Autodesk Inventor part; units mm, degrees
(part 4 of 5)
sketch "Эскиз44" plane through (1.5, 0, 0) normal (1, 0, 0) x (0, 0, -1)
  line L0 (40, 27.152) -> (40, 3) projected
  arc A0 (37, 0) -> (40, 3) centre (37, 3) ccw projected
  line L1 (37, 0) -> (-7, 0) projected
  arc A1 (-10, 3) -> (-7, 0) centre (-7, 3) ccw projected
  line L2 (-10, 3) -> (-10, 160) projected
  arc A2 (-7, 163) -> (-10, 160) centre (-7, 160) ccw projected
  line L3 (-7, 163) -> (37, 163) projected
  arc A3 (40, 160) -> (37, 163) centre (37, 160) ccw projected
  line L4 (40, 160) -> (40, 111.152) projected
  arc A4 (40, 111.152) -> (42, 109.152) centre (42, 111.152) ccw projected
  line L5 (42, 109.152) -> (54, 109.152) projected
  arc A5 (56, 107.152) -> (54, 109.152) centre (54, 107.152) ccw projected
  line L6 (56, 107.152) -> (56, 31.152) projected
  arc A6 (54, 29.152) -> (56, 31.152) centre (54, 31.152) ccw projected
  line L7 (54, 29.152) -> (42, 29.152) projected
  circle A7 centre (383.6, 368.9) radius 1.625 projected
  circle A8 centre (-13.6, 369) radius 1.625 projected
  circle A9 centre (383.6, 1.1) radius 1.625 projected
  circle A10 centre (-13.6, 1.1) radius 1.625 projected
  circle A11 centre (379.0468, 185.0848) radius 1.625 projected
  circle A12 centre (-9.0468, 185.0848) radius 1.625 projected
  circle A13 centre (379, 228) radius 1.625 projected
  circle A14 centre (-9, 228) radius 1.625 projected
  arc A15 (314.8984, 369.1946) -> (314.8984, 366.8054) centre (313.7968, 368) ccw projected
  arc A16 (314.8984, 366.8054) -> (314.8984, 369.1946) centre (316, 368) ccw projected
  arc A17 (297.8984, 229.1946) -> (297.8984, 226.8054) centre (296.7968, 228) ccw projected
  arc A18 (297.8984, 226.8054) -> (297.8984, 229.1946) centre (299, 228) ccw projected
  circle A19 centre (54, 228) radius 1.625 projected
  circle A20 centre (71, 142) radius 1.625 projected
  circle A21 centre (71, 2.0002) radius 1.625 projected
  circle A22 centre (54, 2.0002) radius 1.625 projected
  circle A23 centre (71, 368) radius 1.625 projected
  circle A24 centre (71, 228) radius 1.625 projected
  arc A25 (314.8984, 143.1946) -> (314.8984, 140.8054) centre (313.7968, 142) ccw projected
  arc A26 (314.8984, 140.8054) -> (314.8984, 143.1946) centre (316, 142) ccw projected
  arc A27 (314.8984, 229.1946) -> (314.8984, 226.8054) centre (313.7968, 228) ccw projected
  arc A28 (314.8984, 226.8054) -> (314.8984, 229.1946) centre (316, 228) ccw projected
  circle A29 centre (183.175, 129.0059) radius 1.85 projected
  arc A30 (297.8984, 369.1946) -> (297.8984, 366.8054) centre (296.7968, 368) ccw projected
  arc A31 (297.8984, 366.8054) -> (297.8984, 369.1946) centre (299, 368) ccw projected
  arc A32 (314.8984, 3.1948) -> (314.8984, 0.8056) centre (313.7968, 2.0002) ccw projected
  arc A33 (314.8984, 0.8056) -> (314.8984, 3.1948) centre (316, 2.0002) ccw projected
  circle A34 centre (54, 142) radius 1.625 projected
  circle A35 centre (54, 368) radius 1.625 projected
  arc A36 (297.8984, 3.1948) -> (297.8984, 0.8056) centre (296.7968, 2.0002) ccw projected
  arc A37 (297.8984, 0.8056) -> (297.8984, 3.1948) centre (299, 2.0002) ccw projected
  arc A38 (297.8984, 143.1946) -> (297.8984, 140.8054) centre (296.7968, 142) ccw projected
  arc A39 (297.8984, 140.8054) -> (297.8984, 143.1946) centre (299, 142) ccw projected
  arc A40 (185, 193.309) -> (185, 192.7028) centre (183.175, 193.0059) ccw projected
  line L8 (185, 193.309) -> (185, 192.7028) projected
  line L9 (14.5, 247.5001) -> (35, 247.5001) projected
  arc A41 (38, 244.5001) -> (35, 247.5001) centre (35, 244.5001) ccw projected
  line L10 (38, 244.5001) -> (38, 185.5001) projected
  arc A42 (35, 182.5001) -> (38, 185.5001) centre (35, 185.5001) ccw projected
  line L11 (35, 182.5001) -> (14.5, 182.5001) projected
  arc A43 (11.5, 185.5001) -> (14.5, 182.5001) centre (14.5, 185.5001) ccw projected
  line L12 (11.5, 185.5001) -> (11.5, 244.5001) projected
  arc A44 (14.5, 247.5001) -> (11.5, 244.5001) centre (14.5, 244.5001) ccw projected
  line L13 (358.5, 244.5001) -> (358.5, 185.5001) projected
  arc A45 (355.5, 182.5001) -> (358.5, 185.5001) centre (355.5, 185.5001) ccw projected
  line L14 (355.5, 182.5001) -> (335, 182.5001) projected
  arc A46 (332, 185.5001) -> (335, 182.5001) centre (335, 185.5001) ccw projected
  line L15 (332, 185.5001) -> (332, 244.5001) projected
  arc A47 (335, 247.5001) -> (332, 244.5001) centre (335, 244.5001) ccw projected
  line L16 (335, 247.5001) -> (355.5, 247.5001) projected
  arc A48 (358.5, 244.5001) -> (355.5, 247.5001) centre (355.5, 244.5001) ccw projected
  line L17 (98.825, 226.3849) -> (98.825, 137.3849) projected
  arc A49 (95.825, 134.3849) -> (98.825, 137.3849) centre (95.825, 137.3849) ccw projected
  line L18 (95.825, 134.3849) -> (87.825, 134.3849) projected
  arc A50 (84.825, 137.3849) -> (87.825, 134.3849) centre (87.825, 137.3849) ccw projected
  line L19 (84.825, 137.3849) -> (84.825, 226.3849) projected
  arc A51 (87.825, 229.3849) -> (84.825, 226.3849) centre (87.825, 226.3849) ccw projected
  line L20 (87.825, 229.3849) -> (95.825, 229.3849) projected
  arc A52 (98.825, 226.3849) -> (95.825, 229.3849) centre (95.825, 226.3849) ccw projected
  circle A53 centre (124.375, 129.0059) radius 2 projected
  circle A54 centre (124.375, 193.0059) radius 2 projected
  circle A55 centre (217.25, 312.9941) radius 2.1 projected
  circle A56 centre (152.75, 57.0059) radius 2.1 projected
  circle A57 centre (152.75, 118.0059) radius 2.1 projected
  circle A58 centre (152.75, 312.9941) radius 2.1 projected
  circle A59 centre (217.25, 251.9941) radius 2.1 projected
  circle A60 centre (217.25, 57.0059) radius 2.1 projected
  circle A61 centre (217.25, 118.0059) radius 2.1 projected
  circle A62 centre (152.75, 251.9941) radius 2.1 projected
  line L21 (165, 44) -> (165, 8) projected
  arc A63 (162, 5) -> (165, 8) centre (162, 8) ccw projected
  line L22 (162, 5) -> (96, 5) projected
  arc A64 (93, 8) -> (96, 5) centre (96, 8) ccw projected
  line L23 (93, 8) -> (93, 44) projected
  arc A65 (96, 47) -> (93, 44) centre (96, 44) ccw projected
  line L24 (96, 47) -> (162, 47) projected
  arc A66 (165, 44) -> (162, 47) centre (162, 44) ccw projected
  circle A67 centre (319.1128, 165.0002) radius 2.1 projected
  circle A68 centre (287, 56.343) radius 2.1 projected
  circle A69 centre (50.8872, 165.0002) radius 2.1 projected
  circle A70 centre (173.9908, 56.343) radius 2.1 projected
  circle A71 centre (135.25, 60) radius 2.1 projected
  circle A72 centre (103, 60) radius 2.1 projected
  line L25 (226.25, 270.0041) -> (226.25, 298.657) projected
  arc A73 (228.25, 300.657) -> (226.25, 298.657) centre (228.25, 298.657) ccw projected
  line L26 (228.25, 300.657) -> (268.3252, 300.657) projected
  arc A74 (269.4885, 297.03) -> (268.3252, 300.657) centre (268.3252, 298.657) ccw projected
  line L27 (269.4885, 297.03) -> (229.4132, 268.3772) projected
  arc A75 (226.25, 270.0041) -> (229.4132, 268.3772) centre (228.25, 270.0041) ccw projected
  arc A76 (235.9248, 170.343) -> (234.7615, 166.7161) centre (235.9248, 168.343) ccw projected
  line L28 (235.9248, 170.343) -> (276, 170.343) projected
  arc A77 (278, 168.343) -> (276, 170.343) centre (276, 168.343) ccw projected
  line L29 (278, 168.343) -> (278, 139.6902) projected
  arc A78 (274.8368, 138.0633) -> (278, 139.6902) centre (276, 139.6902) ccw projected
  line L30 (274.8368, 138.0633) -> (234.7615, 166.7161) projected
  arc A79 (94, 106.343) -> (92, 104.343) centre (94, 104.343) ccw projected
  line L31 (94, 106.343) -> (134.0752, 106.343) projected
  arc A80 (135.2385, 102.7161) -> (134.0752, 106.343) centre (134.0752, 104.343) ccw projected
  line L32 (135.2385, 102.7161) -> (95.1632, 74.0633) projected
  arc A81 (92, 75.6902) -> (95.1632, 74.0633) centre (94, 75.6902) ccw projected
  line L33 (92, 75.6902) -> (92, 104.343) projected
  arc A82 (92, 265.657) -> (94, 263.657) centre (94, 265.657) ccw projected
  line L34 (92, 265.657) -> (92, 294.3098) projected
  arc A83 (95.1632, 295.9367) -> (92, 294.3098) centre (94, 294.3098) ccw projected
  line L35 (95.1632, 295.9367) -> (135.2385, 267.2839) projected
  arc A84 (134.0752, 263.657) -> (135.2385, 267.2839) centre (134.0752, 265.657) ccw projected
  line L36 (134.0752, 263.657) -> (94, 263.657) projected
  arc A85 (130.725, 206.0059) -> (132.725, 204.0059) centre (132.725, 206.0059) ccw projected
  line L37 (130.725, 206.0059) -> (130.725, 234.2716) projected
  arc A86 (133.9769, 235.8314) -> (130.725, 234.2716) centre (132.725, 234.2716) ccw projected
  line L38 (133.9769, 235.8314) -> (169.1945, 207.5656) projected
  arc A87 (167.9426, 204.0059) -> (169.1945, 207.5656) centre (167.9426, 206.0059) ccw projected
  line L39 (167.9426, 204.0059) -> (132.725, 204.0059) projected
  arc A88 (226.25, 71.343) -> (228.25, 69.343) centre (228.25, 71.343) ccw projected
  line L40 (226.25, 71.343) -> (226.25, 99.9959) projected
  arc A89 (229.4132, 101.6228) -> (226.25, 99.9959) centre (228.25, 99.9959) ccw projected
  line L41 (229.4132, 101.6228) -> (269.4885, 72.97) projected
  arc A90 (268.3252, 69.343) -> (269.4885, 72.97) centre (268.3252, 71.343) ccw projected
  line L42 (268.3252, 69.343) -> (228.25, 69.343) projected
  arc A91 (226.25, 201.657) -> (228.25, 199.657) centre (228.25, 201.657) ccw projected
  line L43 (226.25, 201.657) -> (226.25, 230.3098) projected
  arc A92 (229.4132, 231.9367) -> (226.25, 230.3098) centre (228.25, 230.3098) ccw projected
  line L44 (229.4132, 231.9367) -> (269.4885, 203.2839) projected
  arc A93 (268.3252, 199.657) -> (269.4885, 203.2839) centre (268.3252, 201.657) ccw projected
  line L45 (268.3252, 199.657) -> (228.25, 199.657) projected
  arc A94 (278, 294.3098) -> (274.8368, 295.9367) centre (276, 294.3098) ccw projected
  line L46 (278, 294.3098) -> (278, 265.657) projected
  arc A95 (276, 263.657) -> (278, 265.657) centre (276, 265.657) ccw projected
  line L47 (276, 263.657) -> (235.9248, 263.657) projected
  arc A96 (234.7615, 267.2839) -> (235.9248, 263.657) centre (235.9248, 265.657) ccw projected
  line L48 (234.7615, 267.2839) -> (274.8368, 295.9367) projected
  arc A97 (226.25, 135.343) -> (228.25, 133.343) centre (228.25, 135.343) ccw projected
  line L49 (226.25, 135.343) -> (226.25, 163.9959) projected
  arc A98 (229.4132, 165.6228) -> (226.25, 163.9959) centre (228.25, 163.9959) ccw projected
  line L50 (229.4132, 165.6228) -> (269.4885, 136.97) projected
  arc A99 (268.3252, 133.343) -> (269.4885, 136.97) centre (268.3252, 135.343) ccw projected
  line L51 (268.3252, 133.343) -> (228.25, 133.343) projected
  arc A100 (143.75, 99.9959) -> (140.5868, 101.6228) centre (141.75, 99.9959) ccw projected
  line L52 (143.75, 99.9959) -> (143.75, 71.343) projected
  arc A101 (141.75, 69.343) -> (143.75, 71.343) centre (141.75, 71.343) ccw projected
  line L53 (141.75, 69.343) -> (101.6748, 69.343) projected
  arc A102 (100.5115, 72.97) -> (101.6748, 69.343) centre (101.6748, 71.343) ccw projected
  line L54 (100.5115, 72.97) -> (140.5868, 101.6228) projected
  arc A103 (143.75, 298.657) -> (141.75, 300.657) centre (141.75, 298.657) ccw projected
  line L55 (143.75, 298.657) -> (143.75, 270.0041) projected
  arc A104 (140.5868, 268.3772) -> (143.75, 270.0041) centre (141.75, 270.0041) ccw projected
  line L56 (140.5868, 268.3772) -> (100.5115, 297.03) projected
  arc A105 (101.6748, 300.657) -> (100.5115, 297.03) centre (101.6748, 298.657) ccw projected
  line L57 (101.6748, 300.657) -> (141.75, 300.657) projected
  line L58 (176.825, 239.0059) -> (176.825, 210.7401) projected
  arc A106 (173.5731, 209.1803) -> (176.825, 210.7401) centre (174.825, 210.7401) ccw projected
  line L59 (173.5731, 209.1803) -> (138.3555, 237.4461) projected
  arc A107 (139.6074, 241.0059) -> (138.3555, 237.4461) centre (139.6074, 239.0059) ccw projected
  line L60 (139.6074, 241.0059) -> (174.825, 241.0059) projected
  arc A108 (176.825, 239.0059) -> (174.825, 241.0059) centre (174.825, 239.0059) ccw projected
  line L61 (278, 104.343) -> (278, 75.6902) projected
  arc A109 (274.8368, 74.0633) -> (278, 75.6902) centre (276, 75.6902) ccw projected
  line L62 (274.8368, 74.0633) -> (234.7615, 102.7161) projected
  arc A110 (235.9248, 106.343) -> (234.7615, 102.7161) centre (235.9248, 104.343) ccw projected
  line L63 (235.9248, 106.343) -> (276, 106.343) projected
  arc A111 (278, 104.343) -> (276, 106.343) centre (276, 104.343) ccw projected
  arc A112 (278, 234.657) -> (276, 236.657) centre (276, 234.657) ccw projected
  line L64 (278, 234.657) -> (278, 206.0041) projected
  arc A113 (274.8368, 204.3772) -> (278, 206.0041) centre (276, 206.0041) ccw projected
  line L65 (274.8368, 204.3772) -> (234.7615, 233.03) projected
  arc A114 (235.9248, 236.657) -> (234.7615, 233.03) centre (235.9248, 234.657) ccw projected
  line L66 (235.9248, 236.657) -> (276, 236.657) projected
  arc A115 (295, 375) -> (292, 372) centre (295, 372) ccw projected
  line L67 (292, 372) -> (292, 323.5966) projected
  arc A116 (289, 320.5966) -> (292, 323.5966) centre (289, 323.5966) ccw projected
  line L68 (289, 320.5966) -> (81, 320.5966) projected
  arc A117 (78, 323.5966) -> (81, 320.5966) centre (81, 323.5966) ccw projected
  line L69 (78, 323.5966) -> (78, 372) projected
  arc A118 (78, 372) -> (75, 375) centre (75, 372) ccw projected
  line L70 (75, 375) -> (-15, 375) projected
  arc A119 (-15, 375) -> (-18, 372) centre (-15, 372) ccw projected
  line L71 (-18, 372) -> (-18, -2) projected
  arc A120 (-18, -2) -> (-15, -5) centre (-15, -2) ccw projected
  line L72 (-15, -5) -> (385, -5) projected
  arc A121 (385, -5) -> (388, -2) centre (385, -2) ccw projected
  line L73 (388, -2) -> (388, 372) projected
  arc A122 (388, 372) -> (385, 375) centre (385, 372) ccw projected
  line L74 (385, 375) -> (295, 375) projected
  line L75 (42, 340.848) -> (54, 340.848) projected
  arc A123 (56, 338.848) -> (54, 340.848) centre (54, 338.848) ccw projected
  line L76 (56, 338.848) -> (56, 262.848) projected
  arc A124 (54, 260.848) -> (56, 262.848) centre (54, 262.848) ccw projected
  line L77 (54, 260.848) -> (-8, 260.848) projected
  arc A125 (-10, 262.848) -> (-8, 260.848) centre (-8, 262.848) ccw projected
  line L78 (-10, 262.848) -> (-10, 367) projected
  arc A126 (-7, 370) -> (-10, 367) centre (-7, 367) ccw projected
  line L79 (-7, 370) -> (37, 370) projected
  arc A127 (40, 367) -> (37, 370) centre (37, 367) ccw projected
  line L80 (40, 367) -> (40, 342.848) projected
  line L81 (377, 0) -> (333, 0) projected
  arc A128 (330, 3) -> (333, 0) centre (333, 3) ccw projected
  line L82 (330, 3) -> (330, 27.152) projected
  line L83 (330, 111.152) -> (330, 160) projected
  arc A129 (333, 163) -> (330, 160) centre (333, 160) ccw projected
  line L84 (333, 163) -> (377, 163) projected
  arc A130 (380, 160) -> (377, 163) centre (377, 160) ccw projected
  line L85 (380, 160) -> (380, 3) projected
  arc A131 (377, 0) -> (380, 3) centre (377, 3) ccw projected
  line L86 (330, 342.848) -> (330, 367) projected
  arc A132 (333, 370) -> (330, 367) centre (333, 367) ccw projected
  line L87 (333, 370) -> (377, 370) projected
  arc A133 (380, 367) -> (377, 370) centre (377, 367) ccw projected
  line L88 (380, 367) -> (380, 262.848) projected
  circle A134 centre (313.7968, 368) radius 1.625
  circle A135 centre (296.7968, 368) radius 1.625
  circle A136 centre (296.7968, 228) radius 1.625
  circle A137 centre (313.7968, 228) radius 1.625
  circle A138 centre (296.7968, 142) radius 1.625
  circle A139 centre (313.7968, 142) radius 1.625
  circle A140 centre (296.7968, 2.0002) radius 1.625
  circle A141 centre (313.7968, 2.0002) radius 1.625
  arc A142 (40, 342.848) -> (42, 340.848) centre (42, 342.848) ccw projected
  arc A143 (42, 29.152) -> (40, 27.152) centre (42, 27.152) ccw projected
  line L89 (316, 109.152) -> (328, 109.152) projected
  line L90 (328, 29.152) -> (316, 29.152) projected
  arc A144 (314, 31.152) -> (316, 29.152) centre (316, 31.152) ccw projected
  line L91 (314, 31.152) -> (314, 107.152) projected
  arc A145 (316, 109.152) -> (314, 107.152) centre (316, 107.152) ccw projected
  line L92 (316, 340.848) -> (328, 340.848) projected
  arc A146 (378, 260.848) -> (380, 262.848) centre (378, 262.848) ccw projected
  line L93 (378, 260.848) -> (316, 260.848) projected
  arc A147 (314, 262.848) -> (316, 260.848) centre (316, 262.848) ccw projected
  line L94 (314, 262.848) -> (314, 338.848) projected
  arc A148 (316, 340.848) -> (314, 338.848) centre (316, 338.848) ccw projected
  arc A149 (330, 27.152) -> (328, 29.152) centre (328, 27.152) ccw projected
  arc A150 (328, 109.152) -> (330, 111.152) centre (328, 111.152) ccw projected
  arc A151 (328, 340.848) -> (330, 342.848) centre (328, 342.848) ccw projected
  point P0 (0, 0)
  point P1 (314.8984, 0.8056)
  point P2 (314.8984, 3.1948)
  point P3 (297.8984, 0.8056)
  point P4 (297.8984, 3.1948)
  point P5 (314.8984, 140.8054)
  point P6 (314.8984, 143.1946)
  point P7 (297.8984, 140.8054)
  point P8 (297.8984, 143.1946)
  point P9 (314.8984, 226.8054)
  point P10 (314.8984, 229.1946)
  point P11 (297.8984, 226.8054)
  point P12 (297.8984, 229.1946)
  point P13 (297.8984, 366.8054)
  point P14 (297.8984, 369.1946)
  point P15 (314.8984, 366.8054)
  point P16 (314.8984, 369.1946)
  constraints: 8 centre point, 1 coincident, 1 concentric
extrude "Выдавливание38" add sketch "Эскиз44" against normal up to surface (1.5 mm away) contours A16 A134 | A18 A136 | A26 A139 | A28 A137 | A31 A135 | A33 A141 | A37 A140 | A39 A138
ref_plane "РабПлоскость2" through (1.5, -2, -185) normal (0, 0, -1) x (-1, 0, 0)
mirror "Зеркальное отражение1" about plane through (1.5, -2, -185) normal (0, 0, -1) of "Выдавливание37"
sketch "Эскиз45" plane through (1.5, 0, 0) normal (1, 0, 0) x (0, 0, -1)
  line L0 (40, 27.152) -> (40, 3) projected
  arc A0 (37, 0) -> (40, 3) centre (37, 3) ccw projected
  line L1 (37, 0) -> (-7, 0) projected
  arc A1 (-10, 3) -> (-7, 0) centre (-7, 3) ccw projected
  line L2 (-10, 3) -> (-10, 160) projected
  arc A2 (-7, 163) -> (-10, 160) centre (-7, 160) ccw projected
  line L3 (-7, 163) -> (37, 163) projected
  arc A3 (40, 160) -> (37, 163) centre (37, 160) ccw projected
  line L4 (40, 160) -> (40, 111.152) projected
  arc A4 (40, 111.152) -> (42, 109.152) centre (42, 111.152) ccw projected
  line L5 (42, 109.152) -> (54, 109.152) projected
  arc A5 (56, 107.152) -> (54, 109.152) centre (54, 107.152) ccw projected
  line L6 (56, 107.152) -> (56, 31.152) projected
  arc A6 (54, 29.152) -> (56, 31.152) centre (54, 31.152) ccw projected
  line L7 (54, 29.152) -> (42, 29.152) projected
  circle A7 centre (383.6, 368.9) radius 1.625 projected
  circle A8 centre (-13.6, 369) radius 1.625 projected
  circle A9 centre (383.6, 1.1) radius 1.625 projected
  circle A10 centre (-13.6, 1.1) radius 1.625 projected
  circle A11 centre (379.0468, 185.0848) radius 1.625 projected
  circle A12 centre (-9.0468, 185.0848) radius 1.625 projected
  circle A13 centre (379, 228) radius 1.625 projected
  circle A14 centre (-9, 228) radius 1.625 projected
  circle A15 centre (313.7968, 368) radius 1.625 projected
  arc A16 (55.1016, 226.8054) -> (55.1016, 229.1946) centre (56.2032, 228) ccw projected
  arc A17 (55.1016, 229.1946) -> (55.1016, 226.8054) centre (54, 228) ccw projected
  arc A18 (72.1016, 140.8054) -> (72.1016, 143.1946) centre (73.2032, 142) ccw projected
  arc A19 (72.1016, 143.1946) -> (72.1016, 140.8054) centre (71, 142) ccw projected
  arc A20 (72.1016, 0.8056) -> (72.1016, 3.1948) centre (73.2032, 2.0002) ccw projected
  arc A21 (72.1016, 3.1948) -> (72.1016, 0.8056) centre (71, 2.0002) ccw projected
  arc A22 (55.1016, 0.8056) -> (55.1016, 3.1948) centre (56.2032, 2.0002) ccw projected
  arc A23 (55.1016, 3.1948) -> (55.1016, 0.8056) centre (54, 2.0002) ccw projected
  arc A24 (72.1016, 366.8054) -> (72.1016, 369.1946) centre (73.2032, 368) ccw projected
  arc A25 (72.1016, 369.1946) -> (72.1016, 366.8054) centre (71, 368) ccw projected
  arc A26 (72.1016, 226.8054) -> (72.1016, 229.1946) centre (73.2032, 228) ccw projected
  arc A27 (72.1016, 229.1946) -> (72.1016, 226.8054) centre (71, 228) ccw projected
  circle A28 centre (183.175, 129.0059) radius 1.85 projected
  circle A29 centre (296.7968, 368) radius 1.625 projected
  circle A30 centre (313.7968, 2.0002) radius 1.625 projected
  arc A31 (55.1016, 140.8054) -> (55.1016, 143.1946) centre (56.2032, 142) ccw projected
  arc A32 (55.1016, 143.1946) -> (55.1016, 140.8054) centre (54, 142) ccw projected
  arc A33 (55.1016, 366.8054) -> (55.1016, 369.1946) centre (56.2032, 368) ccw projected
  arc A34 (55.1016, 369.1946) -> (55.1016, 366.8054) centre (54, 368) ccw projected
  circle A35 centre (296.7968, 2.0002) radius 1.625 projected
  arc A36 (185, 193.309) -> (185, 192.7028) centre (183.175, 193.0059) ccw projected
  line L8 (185, 193.309) -> (185, 192.7028) projected
  line L9 (14.5, 247.5001) -> (35, 247.5001) projected
  arc A37 (38, 244.5001) -> (35, 247.5001) centre (35, 244.5001) ccw projected
  line L10 (38, 244.5001) -> (38, 185.5001) projected
  arc A38 (35, 182.5001) -> (38, 185.5001) centre (35, 185.5001) ccw projected
  line L11 (35, 182.5001) -> (14.5, 182.5001) projected
  arc A39 (11.5, 185.5001) -> (14.5, 182.5001) centre (14.5, 185.5001) ccw projected
  line L12 (11.5, 185.5001) -> (11.5, 244.5001) projected
  arc A40 (14.5, 247.5001) -> (11.5, 244.5001) centre (14.5, 244.5001) ccw projected
  line L13 (358.5, 244.5001) -> (358.5, 185.5001) projected
  arc A41 (355.5, 182.5001) -> (358.5, 185.5001) centre (355.5, 185.5001) ccw projected
  line L14 (355.5, 182.5001) -> (335, 182.5001) projected
  arc A42 (332, 185.5001) -> (335, 182.5001) centre (335, 185.5001) ccw projected
  line L15 (332, 185.5001) -> (332, 244.5001) projected
  arc A43 (335, 247.5001) -> (332, 244.5001) centre (335, 244.5001) ccw projected
  line L16 (335, 247.5001) -> (355.5, 247.5001) projected
  arc A44 (358.5, 244.5001) -> (355.5, 247.5001) centre (355.5, 244.5001) ccw projected
  line L17 (98.825, 226.3849) -> (98.825, 137.3849) projected
  arc A45 (95.825, 134.3849) -> (98.825, 137.3849) centre (95.825, 137.3849) ccw projected
  line L18 (95.825, 134.3849) -> (87.825, 134.3849) projected
  arc A46 (84.825, 137.3849) -> (87.825, 134.3849) centre (87.825, 137.3849) ccw projected
  line L19 (84.825, 137.3849) -> (84.825, 226.3849) projected
  arc A47 (87.825, 229.3849) -> (84.825, 226.3849) centre (87.825, 226.3849) ccw projected
  line L20 (87.825, 229.3849) -> (95.825, 229.3849) projected
  arc A48 (98.825, 226.3849) -> (95.825, 229.3849) centre (95.825, 226.3849) ccw projected
  circle A49 centre (124.375, 129.0059) radius 2 projected
  circle A50 centre (124.375, 193.0059) radius 2 projected
  circle A51 centre (217.25, 312.9941) radius 2.1 projected
  circle A52 centre (152.75, 57.0059) radius 2.1 projected
  circle A53 centre (152.75, 118.0059) radius 2.1 projected
  circle A54 centre (152.75, 312.9941) radius 2.1 projected
  circle A55 centre (217.25, 251.9941) radius 2.1 projected
  circle A56 centre (217.25, 57.0059) radius 2.1 projected
  circle A57 centre (217.25, 118.0059) radius 2.1 projected
  circle A58 centre (152.75, 251.9941) radius 2.1 projected
  line L21 (165, 44) -> (165, 8) projected
  arc A59 (162, 5) -> (165, 8) centre (162, 8) ccw projected
  line L22 (162, 5) -> (96, 5) projected
  arc A60 (93, 8) -> (96, 5) centre (96, 8) ccw projected
  line L23 (93, 8) -> (93, 44) projected
  arc A61 (96, 47) -> (93, 44) centre (96, 44) ccw projected
  line L24 (96, 47) -> (162, 47) projected
  arc A62 (165, 44) -> (162, 47) centre (162, 44) ccw projected
  circle A63 centre (319.1128, 165.0002) radius 2.1 projected
  circle A64 centre (287, 56.343) radius 2.1 projected
  circle A65 centre (50.8872, 165.0002) radius 2.1 projected
  circle A66 centre (173.9908, 56.343) radius 2.1 projected
  circle A67 centre (135.25, 60) radius 2.1 projected
  circle A68 centre (103, 60) radius 2.1 projected
  line L25 (226.25, 270.0041) -> (226.25, 298.657) projected
  arc A69 (228.25, 300.657) -> (226.25, 298.657) centre (228.25, 298.657) ccw projected
  line L26 (228.25, 300.657) -> (268.3252, 300.657) projected
  arc A70 (269.4885, 297.03) -> (268.3252, 300.657) centre (268.3252, 298.657) ccw projected
  line L27 (269.4885, 297.03) -> (229.4132, 268.3772) projected
  arc A71 (226.25, 270.0041) -> (229.4132, 268.3772) centre (228.25, 270.0041) ccw projected
  arc A72 (235.9248, 170.343) -> (234.7615, 166.7161) centre (235.9248, 168.343) ccw projected
  line L28 (235.9248, 170.343) -> (276, 170.343) projected
  arc A73 (278, 168.343) -> (276, 170.343) centre (276, 168.343) ccw projected
  line L29 (278, 168.343) -> (278, 139.6902) projected
  arc A74 (274.8368, 138.0633) -> (278, 139.6902) centre (276, 139.6902) ccw projected
  line L30 (274.8368, 138.0633) -> (234.7615, 166.7161) projected
  arc A75 (94, 106.343) -> (92, 104.343) centre (94, 104.343) ccw projected
  line L31 (94, 106.343) -> (134.0752, 106.343) projected
  arc A76 (135.2385, 102.7161) -> (134.0752, 106.343) centre (134.0752, 104.343) ccw projected
  line L32 (135.2385, 102.7161) -> (95.1632, 74.0633) projected
  arc A77 (92, 75.6902) -> (95.1632, 74.0633) centre (94, 75.6902) ccw projected
  line L33 (92, 75.6902) -> (92, 104.343) projected
  arc A78 (92, 265.657) -> (94, 263.657) centre (94, 265.657) ccw projected
  line L34 (92, 265.657) -> (92, 294.3098) projected
  arc A79 (95.1632, 295.9367) -> (92, 294.3098) centre (94, 294.3098) ccw projected
  line L35 (95.1632, 295.9367) -> (135.2385, 267.2839) projected
  arc A80 (134.0752, 263.657) -> (135.2385, 267.2839) centre (134.0752, 265.657) ccw projected
  line L36 (134.0752, 263.657) -> (94, 263.657) projected
  arc A81 (130.725, 206.0059) -> (132.725, 204.0059) centre (132.725, 206.0059) ccw projected
  line L37 (130.725, 206.0059) -> (130.725, 234.2716) projected
  arc A82 (133.9769, 235.8314) -> (130.725, 234.2716) centre (132.725, 234.2716) ccw projected
  line L38 (133.9769, 235.8314) -> (169.1945, 207.5656) projected
  arc A83 (167.9426, 204.0059) -> (169.1945, 207.5656) centre (167.9426, 206.0059) ccw projected
  line L39 (167.9426, 204.0059) -> (132.725, 204.0059) projected
  arc A84 (226.25, 71.343) -> (228.25, 69.343) centre (228.25, 71.343) ccw projected
  line L40 (226.25, 71.343) -> (226.25, 99.9959) projected
  arc A85 (229.4132, 101.6228) -> (226.25, 99.9959) centre (228.25, 99.9959) ccw projected
  line L41 (229.4132, 101.6228) -> (269.4885, 72.97) projected
  arc A86 (268.3252, 69.343) -> (269.4885, 72.97) centre (268.3252, 71.343) ccw projected
  line L42 (268.3252, 69.343) -> (228.25, 69.343) projected
  arc A87 (226.25, 201.657) -> (228.25, 199.657) centre (228.25, 201.657) ccw projected
  line L43 (226.25, 201.657) -> (226.25, 230.3098) projected
  arc A88 (229.4132, 231.9367) -> (226.25, 230.3098) centre (228.25, 230.3098) ccw projected
  line L44 (229.4132, 231.9367) -> (269.4885, 203.2839) projected
  arc A89 (268.3252, 199.657) -> (269.4885, 203.2839) centre (268.3252, 201.657) ccw projected
  line L45 (268.3252, 199.657) -> (228.25, 199.657) projected
  arc A90 (278, 294.3098) -> (274.8368, 295.9367) centre (276, 294.3098) ccw projected
  line L46 (278, 294.3098) -> (278, 265.657) projected
  arc A91 (276, 263.657) -> (278, 265.657) centre (276, 265.657) ccw projected
  line L47 (276, 263.657) -> (235.9248, 263.657) projected
  arc A92 (234.7615, 267.2839) -> (235.9248, 263.657) centre (235.9248, 265.657) ccw projected
  line L48 (234.7615, 267.2839) -> (274.8368, 295.9367) projected
  arc A93 (226.25, 135.343) -> (228.25, 133.343) centre (228.25, 135.343) ccw projected
  line L49 (226.25, 135.343) -> (226.25, 163.9959) projected
  arc A94 (229.4132, 165.6228) -> (226.25, 163.9959) centre (228.25, 163.9959) ccw projected
  line L50 (229.4132, 165.6228) -> (269.4885, 136.97) projected
  arc A95 (268.3252, 133.343) -> (269.4885, 136.97) centre (268.3252, 135.343) ccw projected
  line L51 (268.3252, 133.343) -> (228.25, 133.343) projected
  arc A96 (143.75, 99.9959) -> (140.5868, 101.6228) centre (141.75, 99.9959) ccw projected
  line L52 (143.75, 99.9959) -> (143.75, 71.343) projected
  arc A97 (141.75, 69.343) -> (143.75, 71.343) centre (141.75, 71.343) ccw projected
  line L53 (141.75, 69.343) -> (101.6748, 69.343) projected
  arc A98 (100.5115, 72.97) -> (101.6748, 69.343) centre (101.6748, 71.343) ccw projected
  line L54 (100.5115, 72.97) -> (140.5868, 101.6228) projected
  arc A99 (143.75, 298.657) -> (141.75, 300.657) centre (141.75, 298.657) ccw projected
  line L55 (143.75, 298.657) -> (143.75, 270.0041) projected
  arc A100 (140.5868, 268.3772) -> (143.75, 270.0041) centre (141.75, 270.0041) ccw projected
  line L56 (140.5868, 268.3772) -> (100.5115, 297.03) projected
  arc A101 (101.6748, 300.657) -> (100.5115, 297.03) centre (101.6748, 298.657) ccw projected
  line L57 (101.6748, 300.657) -> (141.75, 300.657) projected
  line L58 (176.825, 239.0059) -> (176.825, 210.7401) projected
  arc A102 (173.5731, 209.1803) -> (176.825, 210.7401) centre (174.825, 210.7401) ccw projected
  line L59 (173.5731, 209.1803) -> (138.3555, 237.4461) projected
  arc A103 (139.6074, 241.0059) -> (138.3555, 237.4461) centre (139.6074, 239.0059) ccw projected
  line L60 (139.6074, 241.0059) -> (174.825, 241.0059) projected
  arc A104 (176.825, 239.0059) -> (174.825, 241.0059) centre (174.825, 239.0059) ccw projected
  line L61 (278, 104.343) -> (278, 75.6902) projected
  arc A105 (274.8368, 74.0633) -> (278, 75.6902) centre (276, 75.6902) ccw projected
  line L62 (274.8368, 74.0633) -> (234.7615, 102.7161) projected
  arc A106 (235.9248, 106.343) -> (234.7615, 102.7161) centre (235.9248, 104.343) ccw projected
  line L63 (235.9248, 106.343) -> (276, 106.343) projected
  arc A107 (278, 104.343) -> (276, 106.343) centre (276, 104.343) ccw projected
  arc A108 (278, 234.657) -> (276, 236.657) centre (276, 234.657) ccw projected
  line L64 (278, 234.657) -> (278, 206.0041) projected
  arc A109 (274.8368, 204.3772) -> (278, 206.0041) centre (276, 206.0041) ccw projected
  line L65 (274.8368, 204.3772) -> (234.7615, 233.03) projected
  arc A110 (235.9248, 236.657) -> (234.7615, 233.03) centre (235.9248, 234.657) ccw projected
  line L66 (235.9248, 236.657) -> (276, 236.657) projected
  arc A111 (295, 375) -> (292, 372) centre (295, 372) ccw projected
  line L67 (292, 372) -> (292, 323.5966) projected
  arc A112 (289, 320.5966) -> (292, 323.5966) centre (289, 323.5966) ccw projected
  line L68 (289, 320.5966) -> (81, 320.5966) projected
  arc A113 (78, 323.5966) -> (81, 320.5966) centre (81, 323.5966) ccw projected
  line L69 (78, 323.5966) -> (78, 372) projected
  arc A114 (78, 372) -> (75, 375) centre (75, 372) ccw projected
  line L70 (75, 375) -> (-15, 375) projected
  arc A115 (-15, 375) -> (-18, 372) centre (-15, 372) ccw projected
  line L71 (-18, 372) -> (-18, -2) projected
  arc A116 (-18, -2) -> (-15, -5) centre (-15, -2) ccw projected
  line L72 (-15, -5) -> (385, -5) projected
  arc A117 (385, -5) -> (388, -2) centre (385, -2) ccw projected
  line L73 (388, -2) -> (388, 372) projected
  arc A118 (388, 372) -> (385, 375) centre (385, 372) ccw projected
  line L74 (385, 375) -> (295, 375) projected
  line L75 (42, 340.848) -> (54, 340.848) projected
  arc A119 (56, 338.848) -> (54, 340.848) centre (54, 338.848) ccw projected
  line L76 (56, 338.848) -> (56, 262.848) projected
  arc A120 (54, 260.848) -> (56, 262.848) centre (54, 262.848) ccw projected
  line L77 (54, 260.848) -> (-8, 260.848) projected
  arc A121 (-10, 262.848) -> (-8, 260.848) centre (-8, 262.848) ccw projected
  line L78 (-10, 262.848) -> (-10, 367) projected
  arc A122 (-7, 370) -> (-10, 367) centre (-7, 367) ccw projected
  line L79 (-7, 370) -> (37, 370) projected
  arc A123 (40, 367) -> (37, 370) centre (37, 367) ccw projected
  line L80 (40, 367) -> (40, 342.848) projected
  line L81 (377, 0) -> (333, 0) projected
  arc A124 (330, 3) -> (333, 0) centre (333, 3) ccw projected
  line L82 (330, 3) -> (330, 27.152) projected
  line L83 (330, 111.152) -> (330, 160) projected
  arc A125 (333, 163) -> (330, 160) centre (333, 160) ccw projected
  line L84 (333, 163) -> (377, 163) projected
  arc A126 (380, 160) -> (377, 163) centre (377, 160) ccw projected
  line L85 (380, 160) -> (380, 3) projected
  arc A127 (377, 0) -> (380, 3) centre (377, 3) ccw projected
  line L86 (330, 342.848) -> (330, 367) projected
  arc A128 (333, 370) -> (330, 367) centre (333, 367) ccw projected
  line L87 (333, 370) -> (377, 370) projected
  arc A129 (380, 367) -> (377, 370) centre (377, 367) ccw projected
  line L88 (380, 367) -> (380, 262.848) projected
  circle A130 centre (73.2032, 368) radius 1.625
  circle A131 centre (56.2032, 368) radius 1.625
  circle A132 centre (73.2032, 228) radius 1.625
  circle A133 centre (56.2032, 228) radius 1.625
  circle A134 centre (73.2032, 142) radius 1.625
  circle A135 centre (56.2032, 142) radius 1.625
  circle A136 centre (73.2032, 2.0002) radius 1.625
  circle A137 centre (56.2032, 2.0002) radius 1.625
  line L89 (291, 320.5966) -> (291, 375)
  line L90 (291, 375) -> (79, 375)
  line L91 (81, 377) -> (81, 320.5966)
  line L92 (289, 320.5966) -> (81, 320.5966) projected
  line L93 (79, 320.5966) -> (79, 377)
  line L94 (79, 377) -> (293, 377)
  line L95 (293, 377) -> (293, 320.5966)
  arc A138 (40, 342.848) -> (42, 340.848) centre (42, 342.848) ccw projected
  arc A139 (42, 29.152) -> (40, 27.152) centre (42, 27.152) ccw projected
  line L96 (316, 109.152) -> (328, 109.152) projected
  line L97 (328, 29.152) -> (316, 29.152) projected
  arc A140 (314, 31.152) -> (316, 29.152) centre (316, 31.152) ccw projected
  line L98 (314, 31.152) -> (314, 107.152) projected
  arc A141 (316, 109.152) -> (314, 107.152) centre (316, 107.152) ccw projected
  line L99 (316, 340.848) -> (328, 340.848) projected
  arc A142 (378, 260.848) -> (380, 262.848) centre (378, 262.848) ccw projected
  line L100 (378, 260.848) -> (316, 260.848) projected
  arc A143 (314, 262.848) -> (316, 260.848) centre (316, 262.848) ccw projected
  line L101 (314, 262.848) -> (314, 338.848) projected
  arc A144 (316, 340.848) -> (314, 338.848) centre (316, 338.848) ccw projected
  arc A145 (330, 27.152) -> (328, 29.152) centre (328, 27.152) ccw projected
  arc A146 (328, 109.152) -> (330, 111.152) centre (328, 111.152) ccw projected
  arc A147 (328, 340.848) -> (330, 342.848) centre (328, 342.848) ccw projected
  line L102 (289, 320.5966) -> (292, 320.5966)
  line L103 (292, 372) -> (292, 323.5966) projected
  line L104 (292, 320.5966) -> (292, 323.5966)
  line L105 (81, 320.5966) -> (76, 320.5966)
  line L106 (78, 323.5966) -> (78, 320)
  point P0 (0, 0)
  point P1 (72.1016, 0.8056)
  point P2 (72.1016, 3.1948)
  point P3 (55.1016, 0.8056)
  point P4 (55.1016, 3.1948)
  point P5 (72.1016, 140.8054)
  point P6 (72.1016, 143.1946)
  point P7 (55.1016, 140.8054)
  point P8 (55.1016, 143.1946)
  point P9 (55.1016, 226.8054)
  point P10 (55.1016, 229.1946)
  point P11 (72.1016, 226.8054)
  point P12 (72.1016, 229.1946)
  point P13 (55.1016, 366.8054)
  point P14 (55.1016, 369.1946)
  point P15 (72.1016, 369.1946)
  point P16 (81, 375)
  point P17 (78, 347.7983)
  point P18 (291, 321.3605)
  point P19 (79, 321.3605)
  dimension "d244" = 1
  dimension "d247" = 0
  dimension "d248" = 0
  dimension "d250" = 2
  constraints: 20 end point, 7 centre point, 6 point on line, 2 tangent, 1 coincident, 1 midpoint, 1 parallel, 1 perpendicular, 3 other
  measures "d244" distance between parallel lines of L67 L89
  measures "d247" distance between parallel lines of L70 L90
  measures "d248" angle of L69 L91
  measures "d250" distance between parallel lines of L91 L93
extrude "Выдавливание39" add sketch "Эскиз45" against normal up to surface (1.5 mm away) contours A17 A133 | A19 A134 | A21 A136 | A23 A137 | A25 A130 | A27 A132 | A32 A135 | A34 A131 | L25 A69 L26 A70 L27 A71 | L28 A73 L29 A74 L30 A72 | L31 A76 L32 A77 L33 A75 | L34 A79 L35 A80 L36 A78 | L37 A82 L38 A83 L39 A81 | L40 A85 L41 A86 L42 A84 | L43 A88 L44 A89 L45 A87 | L46 A91 L47 A92 L48 A90 | L49 A94 L50 A95 L51 A93 | L52 A97 L53 A98 L54 A96 | L55 A100 L56 A101 L57 A99 | L58 A102 L59 A103 L60 A104 | L61 A105 L62 A106 L63 A107 | L64 A109 L65 A110 L66 A108 | A112 L68 L91 L90 L89 | L91 A113 L93 L90
sketch "Эскиз46" plane through (1.5, 0, 0) normal (1, 0, 0) x (0, 0, -1)
  line L0 (289, 320.5966) -> (81, 320.5966) projected
  line L1 (79, 320.5966) -> (291, 320.5966)
  line L2 (291, 320.5966) -> (291, 375)
  line L3 (291, 375) -> (79, 375)
  line L4 (79, 375) -> (79, 320.5966)
  line L5 (40, 27.152) -> (40, 3) projected
  arc A0 (37, 0) -> (40, 3) centre (37, 3) ccw projected
  line L6 (37, 0) -> (-7, 0) projected
  arc A1 (-10, 3) -> (-7, 0) centre (-7, 3) ccw projected
  line L7 (-10, 3) -> (-10, 160) projected
  arc A2 (-7, 163) -> (-10, 160) centre (-7, 160) ccw projected
  line L8 (-7, 163) -> (37, 163) projected
  arc A3 (40, 160) -> (37, 163) centre (37, 160) ccw projected
  line L9 (40, 160) -> (40, 111.152) projected
  arc A4 (40, 111.152) -> (42, 109.152) centre (42, 111.152) ccw projected
  line L10 (42, 109.152) -> (54, 109.152) projected
  arc A5 (56, 107.152) -> (54, 109.152) centre (54, 107.152) ccw projected
  line L11 (56, 107.152) -> (56, 31.152) projected
  arc A6 (54, 29.152) -> (56, 31.152) centre (54, 31.152) ccw projected
  line L12 (54, 29.152) -> (42, 29.152) projected
  circle A7 centre (383.6, 368.9) radius 1.625 projected
  circle A8 centre (-13.6, 369) radius 1.625 projected
  circle A9 centre (383.6, 1.1) radius 1.625 projected
  circle A10 centre (-13.6, 1.1) radius 1.625 projected
  circle A11 centre (379.0468, 185.0848) radius 1.625 projected
  circle A12 centre (-9.0468, 185.0848) radius 1.625 projected
  circle A13 centre (379, 228) radius 1.625 projected
  circle A14 centre (-9, 228) radius 1.625 projected
  circle A15 centre (313.7968, 368) radius 1.625 projected
  circle A16 centre (73.2032, 142) radius 1.625 projected
  circle A17 centre (73.2032, 2.0002) radius 1.625 projected
  circle A18 centre (56.2032, 2.0002) radius 1.625 projected
  circle A19 centre (183.175, 129.0059) radius 1.85 projected
  circle A20 centre (296.7968, 368) radius 1.625 projected
  circle A21 centre (313.7968, 2.0002) radius 1.625 projected
  circle A22 centre (56.2032, 142) radius 1.625 projected
  circle A23 centre (296.7968, 2.0002) radius 1.625 projected
  arc A24 (185, 193.309) -> (185, 192.7028) centre (183.175, 193.0059) ccw projected
  line L13 (185, 193.309) -> (185, 192.7028) projected
  line L14 (14.5, 247.5001) -> (35, 247.5001) projected
  arc A25 (38, 244.5001) -> (35, 247.5001) centre (35, 244.5001) ccw projected
  line L15 (38, 244.5001) -> (38, 185.5001) projected
  arc A26 (35, 182.5001) -> (38, 185.5001) centre (35, 185.5001) ccw projected
  line L16 (35, 182.5001) -> (14.5, 182.5001) projected
  arc A27 (11.5, 185.5001) -> (14.5, 182.5001) centre (14.5, 185.5001) ccw projected
  line L17 (11.5, 185.5001) -> (11.5, 244.5001) projected
  arc A28 (14.5, 247.5001) -> (11.5, 244.5001) centre (14.5, 244.5001) ccw projected
  line L18 (358.5, 244.5001) -> (358.5, 185.5001) projected
  arc A29 (355.5, 182.5001) -> (358.5, 185.5001) centre (355.5, 185.5001) ccw projected
  line L19 (355.5, 182.5001) -> (335, 182.5001) projected
  arc A30 (332, 185.5001) -> (335, 182.5001) centre (335, 185.5001) ccw projected
  line L20 (332, 185.5001) -> (332, 244.5001) projected
  arc A31 (335, 247.5001) -> (332, 244.5001) centre (335, 244.5001) ccw projected
  line L21 (335, 247.5001) -> (355.5, 247.5001) projected
  arc A32 (358.5, 244.5001) -> (355.5, 247.5001) centre (355.5, 244.5001) ccw projected
  line L22 (98.825, 226.3849) -> (98.825, 137.3849) projected
  arc A33 (95.825, 134.3849) -> (98.825, 137.3849) centre (95.825, 137.3849) ccw projected
  line L23 (95.825, 134.3849) -> (87.825, 134.3849) projected
  arc A34 (84.825, 137.3849) -> (87.825, 134.3849) centre (87.825, 137.3849) ccw projected
  line L24 (84.825, 137.3849) -> (84.825, 226.3849) projected
  arc A35 (87.825, 229.3849) -> (84.825, 226.3849) centre (87.825, 226.3849) ccw projected
  line L25 (87.825, 229.3849) -> (95.825, 229.3849) projected
  arc A36 (98.825, 226.3849) -> (95.825, 229.3849) centre (95.825, 226.3849) ccw projected
  circle A37 centre (124.375, 129.0059) radius 2 projected
  circle A38 centre (124.375, 193.0059) radius 2 projected
  circle A39 centre (217.25, 312.9941) radius 2.1 projected
  circle A40 centre (152.75, 57.0059) radius 2.1 projected
  circle A41 centre (152.75, 118.0059) radius 2.1 projected
  circle A42 centre (152.75, 312.9941) radius 2.1 projected
  circle A43 centre (217.25, 251.9941) radius 2.1 projected
  circle A44 centre (217.25, 57.0059) radius 2.1 projected
  circle A45 centre (217.25, 118.0059) radius 2.1 projected
  circle A46 centre (152.75, 251.9941) radius 2.1 projected
  line L26 (165, 44) -> (165, 8) projected
  arc A47 (162, 5) -> (165, 8) centre (162, 8) ccw projected
  line L27 (162, 5) -> (96, 5) projected
  arc A48 (93, 8) -> (96, 5) centre (96, 8) ccw projected
  line L28 (93, 8) -> (93, 44) projected
  arc A49 (96, 47) -> (93, 44) centre (96, 44) ccw projected
  line L29 (96, 47) -> (162, 47) projected
  arc A50 (165, 44) -> (162, 47) centre (162, 44) ccw projected
  circle A51 centre (319.1128, 165.0002) radius 2.1 projected
  circle A52 centre (287, 56.343) radius 2.1 projected
  circle A53 centre (50.8872, 165.0002) radius 2.1 projected
  circle A54 centre (173.9908, 56.343) radius 2.1 projected
  circle A55 centre (135.25, 60) radius 2.1 projected
  circle A56 centre (103, 60) radius 2.1 projected
  arc A57 (295, 375) -> (292, 372) centre (295, 372) ccw projected
  line L30 (292, 372) -> (292, 323.5966) projected
  arc A58 (291, 321.3605) -> (292, 323.5966) centre (289, 323.5966) ccw projected
  arc A59 (78, 323.5966) -> (79, 321.3605) centre (81, 323.5966) ccw projected
  line L31 (78, 323.5966) -> (78, 372) projected
  arc A60 (78, 372) -> (75, 375) centre (75, 372) ccw projected
  line L32 (75, 375) -> (-15, 375) projected
  arc A61 (-15, 375) -> (-18, 372) centre (-15, 372) ccw projected
  line L33 (-18, 372) -> (-18, -2) projected
  arc A62 (-18, -2) -> (-15, -5) centre (-15, -2) ccw projected
  line L34 (-15, -5) -> (385, -5) projected
  arc A63 (385, -5) -> (388, -2) centre (385, -2) ccw projected
  line L35 (388, -2) -> (388, 372) projected
  arc A64 (388, 372) -> (385, 375) centre (385, 372) ccw projected
  line L36 (385, 375) -> (295, 375) projected
  line L37 (42, 340.848) -> (54, 340.848) projected
  arc A65 (56, 338.848) -> (54, 340.848) centre (54, 338.848) ccw projected
  line L38 (56, 338.848) -> (56, 262.848) projected
  arc A66 (54, 260.848) -> (56, 262.848) centre (54, 262.848) ccw projected
  line L39 (54, 260.848) -> (-8, 260.848) projected
  arc A67 (-10, 262.848) -> (-8, 260.848) centre (-8, 262.848) ccw projected
  line L40 (-10, 262.848) -> (-10, 367) projected
  arc A68 (-7, 370) -> (-10, 367) centre (-7, 367) ccw projected
  line L41 (-7, 370) -> (37, 370) projected
  arc A69 (40, 367) -> (37, 370) centre (37, 367) ccw projected
  line L42 (40, 367) -> (40, 342.848) projected
  line L43 (377, 0) -> (333, 0) projected
  arc A70 (330, 3) -> (333, 0) centre (333, 3) ccw projected
  line L44 (330, 3) -> (330, 27.152) projected
  line L45 (330, 111.152) -> (330, 160) projected
  arc A71 (333, 163) -> (330, 160) centre (333, 160) ccw projected
  line L46 (333, 163) -> (377, 163) projected
  arc A72 (380, 160) -> (377, 163) centre (377, 160) ccw projected
  line L47 (380, 160) -> (380, 3) projected
  arc A73 (377, 0) -> (380, 3) centre (377, 3) ccw projected
  line L48 (330, 342.848) -> (330, 367) projected
  arc A74 (333, 370) -> (330, 367) centre (333, 367) ccw projected
  line L49 (333, 370) -> (377, 370) projected
  arc A75 (380, 367) -> (377, 370) centre (377, 367) ccw projected
  line L50 (380, 367) -> (380, 262.848) projected
  line L51 (73.2032, 142) -> (79.2032, 142)
  line L52 (87.825, 134.3849) -> (78.75, 134.3849)
  line L53 (78.75, 134.3849) -> (78.75, 229.3849)
  line L54 (78.75, 229.3849) -> (87.825, 229.3849)
  line L55 (87.825, 229.3849) -> (87.825, 134.3849)
  line L56 (95.825, 134.3849) -> (100.825, 134.3849)
  line L57 (100.825, 134.3849) -> (100.825, 229.3849)
  line L58 (100.825, 229.3849) -> (95.825, 229.3849)
  line L59 (95.825, 229.3849) -> (95.825, 134.3849)
  line L60 (291, 321.3605) -> (291, 375) projected
  line L61 (291, 375) -> (79, 375) projected
  line L62 (79, 375) -> (79, 321.3605) projected
  arc A76 (40, 342.848) -> (42, 340.848) centre (42, 342.848) ccw projected
  arc A77 (42, 29.152) -> (40, 27.152) centre (42, 27.152) ccw projected
  line L63 (316, 109.152) -> (328, 109.152) projected
  line L64 (328, 29.152) -> (316, 29.152) projected
  arc A78 (314, 31.152) -> (316, 29.152) centre (316, 31.152) ccw projected
  line L65 (314, 31.152) -> (314, 107.152) projected
  arc A79 (316, 109.152) -> (314, 107.152) centre (316, 107.152) ccw projected
  line L66 (316, 340.848) -> (328, 340.848) projected
  arc A80 (378, 260.848) -> (380, 262.848) centre (378, 262.848) ccw projected
  line L67 (378, 260.848) -> (316, 260.848) projected
  arc A81 (314, 262.848) -> (316, 260.848) centre (316, 262.848) ccw projected
  line L68 (314, 262.848) -> (314, 338.848) projected
  arc A82 (316, 340.848) -> (314, 338.848) centre (316, 338.848) ccw projected
  arc A83 (330, 27.152) -> (328, 29.152) centre (328, 27.152) ccw projected
  arc A84 (328, 109.152) -> (330, 111.152) centre (328, 111.152) ccw projected
  arc A85 (328, 340.848) -> (330, 342.848) centre (328, 342.848) ccw projected
  line L69 (292, 323.5966) -> (292, 320.5966)
  line L70 (292, 320.5966) -> (291, 320.5966)
  line L71 (78, 323.5966) -> (78, 320.5966)
  line L72 (78, 320.5966) -> (79, 320.5966)
  point P0 (0, 0)
  point P1 (291, 321.3605)
  dimension "d237" = 0
  dimension "d238" = 1
  dimension "d239" = 1
  dimension "d240" = 6
  dimension "d241" = 5
  constraints: 34 end point, 6 parallel, 5 perpendicular, 4 horizontal, 4 point on line, 1 collinear, 1 point on circle, 1 tangent, 1 vertical
  measures "d237" distance between parallel lines of L32 L3
  measures "d238" distance between parallel lines of L31 L4
  measures "d239" distance between parallel lines of L30 L2
  measures "d240" distance of L51.start L51.end
  measures "d241" distance of L58.end L57.end
extrude "Выдавливание40" cut sketch "Эскиз46" against normal blind 10 contours L2 A58 L69 L70 | L72 L71 A59 L4 | A36 L58 L57 L56 A33 L22 | L22 A33 L59 A36 | L59 L23 L55 L25 | L55 A34 L24 A35 | A35 L24 A34 L52 L53 L54
fillet "Сопряжение4" radius 2 2 edges at (0.75, 375, -79) (0.75, 375, -291)
sketch "Эскиз47" plane through (1.5, 0, 0) normal (1, 0, 0) x (0, 0, -1)
  arc A0 (291, 373) -> (289, 375) centre (289, 373) ccw projected
  line L0 (289, 375) -> (81, 375) projected
  arc A1 (81, 375) -> (79, 373) centre (81, 373) ccw projected
  line L1 (78, 320.5966) -> (78, 372) projected
  arc A2 (78, 372) -> (75, 375) centre (75, 372) ccw projected
  line L2 (75, 375) -> (-15, 375) projected
  arc A3 (-15, 375) -> (-18, 372) centre (-15, 372) ccw projected
  line L3 (-18, 372) -> (-18, -2) projected
  arc A4 (-18, -2) -> (-15, -5) centre (-15, -2) ccw projected
  line L4 (-15, -5) -> (385, -5) projected
  arc A5 (385, -5) -> (388, -2) centre (385, -2) ccw projected
  line L5 (388, -2) -> (388, 372) projected
  arc A6 (388, 372) -> (385, 375) centre (385, 372) ccw projected
  line L6 (385, 375) -> (295, 375) projected
  arc A7 (295, 375) -> (292, 372) centre (295, 372) ccw projected
  line L7 (292, 372) -> (292, 320.5966) projected
  line L8 (100.825, 134.3849) -> (78.75, 134.3849) projected
  line L9 (78.75, 134.3849) -> (78.75, 229.3849) projected
  line L10 (78.75, 229.3849) -> (100.825, 229.3849) projected
  line L11 (100.825, 229.3849) -> (100.825, 134.3849) projected
  line L12 (40, 27.152) -> (40, 3) projected
  arc A8 (37, 0) -> (40, 3) centre (37, 3) ccw projected
  line L13 (37, 0) -> (-7, 0) projected
  arc A9 (-10, 3) -> (-7, 0) centre (-7, 3) ccw projected
  line L14 (-10, 3) -> (-10, 160) projected
  arc A10 (-7, 163) -> (-10, 160) centre (-7, 160) ccw projected
  line L15 (-7, 163) -> (37, 163) projected
  arc A11 (40, 160) -> (37, 163) centre (37, 160) ccw projected
  line L16 (40, 160) -> (40, 111.152) projected
  arc A12 (40, 111.152) -> (42, 109.152) centre (42, 111.152) ccw projected
  line L17 (42, 109.152) -> (54, 109.152) projected
  arc A13 (56, 107.152) -> (54, 109.152) centre (54, 107.152) ccw projected
  line L18 (56, 107.152) -> (56, 31.152) projected
  arc A14 (54, 29.152) -> (56, 31.152) centre (54, 31.152) ccw projected
  line L19 (54, 29.152) -> (42, 29.152) projected
  circle A15 centre (383.6, 368.9) radius 1.625 projected
  circle A16 centre (-13.6, 369) radius 1.625 projected
  circle A17 centre (383.6, 1.1) radius 1.625 projected
  circle A18 centre (-13.6, 1.1) radius 1.625 projected
  circle A19 centre (379.0468, 185.0848) radius 1.625 projected
  circle A20 centre (-9.0468, 185.0848) radius 1.625 projected
  circle A21 centre (379, 228) radius 1.625 projected
  circle A22 centre (-9, 228) radius 1.625 projected
  circle A23 centre (313.7968, 368) radius 1.625 projected
  circle A24 centre (73.2032, 142) radius 1.625 projected
  circle A25 centre (73.2032, 2.0002) radius 1.625 projected
  circle A26 centre (56.2032, 2.0002) radius 1.625 projected
  circle A27 centre (183.175, 129.0059) radius 1.85 projected
  circle A28 centre (296.7968, 368) radius 1.625 projected
  circle A29 centre (313.7968, 2.0002) radius 1.625 projected
  circle A30 centre (56.2032, 142) radius 1.625 projected
  circle A31 centre (296.7968, 2.0002) radius 1.625 projected
  arc A32 (185, 193.309) -> (185, 192.7028) centre (183.175, 193.0059) ccw projected
  line L20 (185, 193.309) -> (185, 192.7028) projected
  line L21 (14.5, 247.5001) -> (35, 247.5001) projected
  arc A33 (38, 244.5001) -> (35, 247.5001) centre (35, 244.5001) ccw projected
  line L22 (38, 244.5001) -> (38, 185.5001) projected
  arc A34 (35, 182.5001) -> (38, 185.5001) centre (35, 185.5001) ccw projected
  line L23 (35, 182.5001) -> (14.5, 182.5001) projected
  arc A35 (11.5, 185.5001) -> (14.5, 182.5001) centre (14.5, 185.5001) ccw projected
  line L24 (11.5, 185.5001) -> (11.5, 244.5001) projected
  arc A36 (14.5, 247.5001) -> (11.5, 244.5001) centre (14.5, 244.5001) ccw projected
  line L25 (358.5, 244.5001) -> (358.5, 185.5001) projected
  arc A37 (355.5, 182.5001) -> (358.5, 185.5001) centre (355.5, 185.5001) ccw projected
  line L26 (355.5, 182.5001) -> (335, 182.5001) projected
  arc A38 (332, 185.5001) -> (335, 182.5001) centre (335, 185.5001) ccw projected
  line L27 (332, 185.5001) -> (332, 244.5001) projected
  arc A39 (335, 247.5001) -> (332, 244.5001) centre (335, 244.5001) ccw projected
  line L28 (335, 247.5001) -> (355.5, 247.5001) projected
  arc A40 (358.5, 244.5001) -> (355.5, 247.5001) centre (355.5, 244.5001) ccw projected
  circle A41 centre (124.375, 129.0059) radius 2 projected
  circle A42 centre (124.375, 193.0059) radius 2 projected
  circle A43 centre (217.25, 312.9941) radius 2.1 projected
  circle A44 centre (152.75, 57.0059) radius 2.1 projected
  circle A45 centre (152.75, 118.0059) radius 2.1 projected
  circle A46 centre (152.75, 312.9941) radius 2.1 projected
  circle A47 centre (217.25, 251.9941) radius 2.1 projected
  circle A48 centre (217.25, 57.0059) radius 2.1 projected
  circle A49 centre (217.25, 118.0059) radius 2.1 projected
  circle A50 centre (152.75, 251.9941) radius 2.1 projected
  line L29 (165, 44) -> (165, 8) projected
  arc A51 (162, 5) -> (165, 8) centre (162, 8) ccw projected
  line L30 (162, 5) -> (96, 5) projected
  arc A52 (93, 8) -> (96, 5) centre (96, 8) ccw projected
  line L31 (93, 8) -> (93, 44) projected
  arc A53 (96, 47) -> (93, 44) centre (96, 44) ccw projected
  line L32 (96, 47) -> (162, 47) projected
  arc A54 (165, 44) -> (162, 47) centre (162, 44) ccw projected
  circle A55 centre (319.1128, 165.0002) radius 2.1 projected
  circle A56 centre (287, 56.343) radius 2.1 projected
  circle A57 centre (50.8872, 165.0002) radius 2.1 projected
  circle A58 centre (173.9908, 56.343) radius 2.1 projected
  circle A59 centre (135.25, 60) radius 2.1 projected
  circle A60 centre (103, 60) radius 2.1 projected
  line L33 (42, 340.848) -> (54, 340.848) projected
  arc A61 (56, 338.848) -> (54, 340.848) centre (54, 338.848) ccw projected
  line L34 (56, 338.848) -> (56, 262.848) projected
  arc A62 (54, 260.848) -> (56, 262.848) centre (54, 262.848) ccw projected
  line L35 (54, 260.848) -> (-8, 260.848) projected
  arc A63 (-10, 262.848) -> (-8, 260.848) centre (-8, 262.848) ccw projected
  line L36 (-10, 262.848) -> (-10, 367) projected
  arc A64 (-7, 370) -> (-10, 367) centre (-7, 367) ccw projected
  line L37 (-7, 370) -> (37, 370) projected
  arc A65 (40, 367) -> (37, 370) centre (37, 367) ccw projected
  line L38 (40, 367) -> (40, 342.848) projected
  line L39 (377, 0) -> (333, 0) projected
  arc A66 (330, 3) -> (333, 0) centre (333, 3) ccw projected
  line L40 (330, 3) -> (330, 27.152) projected
  line L41 (330, 111.152) -> (330, 160) projected
  arc A67 (333, 163) -> (330, 160) centre (333, 160) ccw projected
  line L42 (333, 163) -> (377, 163) projected
  arc A68 (380, 160) -> (377, 163) centre (377, 160) ccw projected
  line L43 (380, 160) -> (380, 3) projected
  arc A69 (377, 0) -> (380, 3) centre (377, 3) ccw projected
  line L44 (330, 342.848) -> (330, 367) projected
  arc A70 (333, 370) -> (330, 367) centre (333, 367) ccw projected
  line L45 (333, 370) -> (377, 370) projected
  arc A71 (380, 367) -> (377, 370) centre (377, 367) ccw projected
  line L46 (380, 367) -> (380, 262.848) projected
  line L47 (296.7968, 2.0002) -> (296.7968, 368)
  line L48 (296.7968, 368) -> (73.2032, 368)
  line L49 (73.2032, 368) -> (73.2032, 2.0002)
  line L50 (73.2032, 2.0002) -> (296.7968, 2.0002)
  line L51 (81.2032, 10.0002) -> (81.2032, 360)
  line L52 (81.2032, 360) -> (288.7968, 360)
  line L53 (288.7968, 360) -> (288.7968, 10.0002)
  line L54 (288.7968, 10.0002) -> (81.2032, 10.0002)
  line L55 (124.375, 129.0059) -> (183.175, 193.0059)
  line L56 (183.175, 193.0059) -> (217.25, 118.0059)
  line L57 (124.375, 193.0059) -> (217.25, 118.0059)
  line L58 (124.375, 129.0059) -> (124.375, 193.0059)
  line L59 (124.375, 193.0059) -> (183.175, 193.0059)
  line L60 (152.75, 251.9941) -> (183.175, 193.0059)
  line L61 (124.375, 193.0059) -> (152.75, 251.9941)
  line L62 (152.75, 251.9941) -> (217.25, 251.9941)
  line L63 (217.25, 251.9941) -> (152.75, 312.9941)
  line L64 (152.75, 312.9941) -> (217.25, 312.9941)
  line L65 (217.25, 312.9941) -> (217.25, 251.9941)
  line L66 (152.75, 251.9941) -> (152.75, 312.9941)
  line L67 (124.375, 193.0059) -> (152.75, 312.9941)
  line L68 (217.25, 118.0059) -> (217.25, 251.9941)
  line L69 (183.175, 193.0059) -> (217.25, 251.9941)
  line L70 (183.175, 129.0059) -> (217.25, 118.0059)
  line L71 (183.175, 129.0059) -> (183.175, 193.0059)
  line L72 (183.175, 129.0059) -> (124.375, 129.0059)
  line L73 (183.175, 129.0059) -> (152.75, 118.0059)
  line L74 (124.375, 129.0059) -> (152.75, 118.0059)
  line L75 (152.75, 118.0059) -> (217.25, 118.0059)
  line L76 (135.25, 60) -> (103, 60)
  line L77 (124.375, 129.0059) -> (103, 60)
  line L78 (217.25, 57.0059) -> (124.375, 129.0059)
  line L79 (124.375, 129.0059) -> (152.75, 57.0059)
  line L80 (217.25, 57.0059) -> (217.25, 118.0059)
  line L81 (135.25, 60) -> (152.75, 57.0059)
  line L82 (173.9908, 56.343) -> (152.75, 57.0059)
  line L83 (152.75, 57.0059) -> (152.75, 118.0059)
  line L84 (173.9908, 56.343) -> (217.25, 57.0059)
  line L85 (173.9908, 56.343) -> (152.75, 118.0059)
  line L86 (135.25, 60) -> (124.375, 129.0059)
  arc A72 (40, 342.848) -> (42, 340.848) centre (42, 342.848) ccw projected
  arc A73 (42, 29.152) -> (40, 27.152) centre (42, 27.152) ccw projected
  line L87 (316, 109.152) -> (328, 109.152) projected
  line L88 (328, 29.152) -> (316, 29.152) projected
  arc A74 (314, 31.152) -> (316, 29.152) centre (316, 31.152) ccw projected
  line L89 (314, 31.152) -> (314, 107.152) projected
  arc A75 (316, 109.152) -> (314, 107.152) centre (316, 107.152) ccw projected
  line L90 (316, 340.848) -> (328, 340.848) projected
  arc A76 (378, 260.848) -> (380, 262.848) centre (378, 262.848) ccw projected
  line L91 (378, 260.848) -> (316, 260.848) projected
  arc A77 (314, 262.848) -> (316, 260.848) centre (316, 262.848) ccw projected
  line L92 (314, 262.848) -> (314, 338.848) projected
  arc A78 (316, 340.848) -> (314, 338.848) centre (316, 338.848) ccw projected
  arc A79 (330, 27.152) -> (328, 29.152) centre (328, 27.152) ccw projected
  arc A80 (328, 109.152) -> (330, 111.152) centre (328, 111.152) ccw projected
  arc A81 (328, 340.848) -> (330, 342.848) centre (328, 342.848) ccw projected
  line L93 (79, 373) -> (79, 320.5966) projected
  line L94 (79, 320.5966) -> (78, 320.5966) projected
  line L95 (292, 320.5966) -> (291, 320.5966) projected
  line L96 (291, 320.5966) -> (291, 373) projected
  point P0 (0, 0)
  dimension "d252" = 8
  constraints: 80 end point, 8 perpendicular, 6 parallel, 4 vertical, 1 horizontal, 3 other
  measures "d252" distance between parallel lines of L49 L51